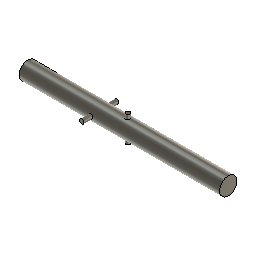
Eixo c um furo v2 (Autodesk Fusion 360 design; units mm, degrees)
Autodesk Fusion 360 part; units mm, degrees
note: some values were not read from the file. Set by a fixed rule: which sketch regions a step uses.
sketch "Esboço1" plane through (0, 0, 0) normal (1, 0, 0) x (0, 1, 0)
  circle A0 centre (0, 0) radius 4
  line L0 (0, 0) -> (3, 0) construction
  line L1 (3, 0) -> (3, -2.6458)
  line L2 (3, 0) -> (3, 2.6458)
  dimension "d1" = 8
  dimension "d2" = 3
  constraint coincident A0.centre L0.start
  constraint horizontal L0
  constraint coincident A0 L1.end
  constraint perpendicular L0 L1
  constraint coincident A0 L2.end
  constraint perpendicular L0 L2
  measures "d1" diameter of A0
  measures "d2" distance of A0.centre L0.end
extrude "Extrusão1" add sketch "Esboço1" along normal blind 92
extrude "Extrusão2" cut sketch "Esboço1" along normal blind 10 contours A0 L1 L2 picked at (3.6528, 0.1921)
sketch "Esboço2" plane through (0, 0, 0) normal (0, 1, 0) x (1, 0, 0)
sketch "Esboço3" plane through (0, 0, 0) normal (0, 0, 1) x (1, 0, 0)
  line L0 (0, 0) -> (46, 0) construction
  circle A0 centre (46, 0) radius 1
  dimension "d7" = 46
  dimension "d24" = 2
  constraint coincident L0.start origin
  constraint horizontal L0
  constraint coincident L0.end A0.centre
  measures "d7" distance of L0.start L0.end
  measures "d24" diameter of A0
sketch "Esboço4" plane through (0, 0, 0) normal (0, 1, 0) x (1, 0, 0)
  line L0 (92, 0) -> (32.816, 0) construction
  circle A0 centre (32.816, 0) radius 1
  dimension "d13" = 59.184
  dimension "d23" = 2
  constraint horizontal L0
  constraint coincident L0.end A0.centre
  measures "d13" distance of L0.start L0.end
  measures "d23" diameter of A0
extrude "Extrusão7" add sketch "Esboço3" along normal blind 6 and the other way blind 6
extrude "Extrusão8" add sketch "Esboço4" along normal blind 7 and the other way blind 7
extrude "Extrusão9" add 1 faces at (32.4233, -7, 0.2267) along direction (0, -1, 0) blind 1
extrude "Extrusão10" add 1 faces at (32.4233, 7, 0.2267) along direction (0, 1, 0) blind 1
sketch "Esboço5" plane through (0, -8, 0) normal (0, -1, 0) x (1, 0, 0)
  circle A0 centre (32.816, 0) radius 1
equation "d13 = 58.434 mm + 0.75 mm"
